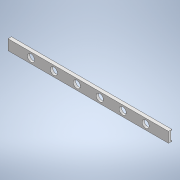
# Autodesk Inventor part: couvercle
Saved by Autodesk Inventor 2020 (Build 240168000, 168)
## iProperties
Created: 2023-04-05
Part Number: couvercle
Material: Générique
Document SubType Name: Modeling
Designer: Admin
Density: 1 g/cm^3
Appearance: Par défaut
Author: Admin
Autodesk Inventor part; units mm, degrees
ref_plane "YZ Plane" through (0, 0, 0) normal (1, 0, 0) x (0, 1, 0)
ref_plane "XZ Plane" through (0, 0, 0) normal (0, 1, 0) x (-1, 0, 0)
ref_plane "XY Plane" through (0, 0, 0) normal (0, 0, 1) x (1, 0, 0)
sketch "Esquisse1" plane through (0, 0, 0) normal (0, 0, 1) x (1, 0, 0)
  line L0 (40, 3.9877) -> (-100, 3.9877)
  line L1 (-100, 3.9877) -> (-100, -4.0123)
  line L2 (-100, -4.0123) -> (40, -4.0123)
  line L3 (40, -4.0123) -> (40, 3.9877)
  circle A0 centre (0, 0) radius 3.125
  line L4 (15.1704, 0) -> (0, 0) construction
  circle A1 centre (-20, 0) radius 3.125
  circle A2 centre (-40, 0) radius 3.125
  circle A3 centre (-60, 0) radius 3.125
  circle A4 centre (-80, 0) radius 3.125
  circle A5 centre (20, 0) radius 3.125
  dimension "d0" = 8
  dimension "d1" = 140
  dimension "d2" = 40
  dimension "d3" = 6.25
  dimension "d6" = 20
  dimension "d13" = 20
  constraints: 10 end point, 6 centre point, 4 horizontal, 2 parallel, 1 coincident, 1 perpendicular, 10 other
  measures "d0" distance of L0.end L1.end
  measures "d1" distance of L1.end L2.end
  measures "d2" distance from line of point (0, 0) L3
  measures "d3" diameter of A0
  measures "d6" distance of L4.end A1.centre
  measures "d13" distance of L4.end A5.centre
extrude "Extrusion1" add sketch "Esquisse1" along normal blind 2
sketch "Esquisse2" plane through (0, 0, 2) normal (0, 0, 1) x (1, 0, 0)
  line L0 (-100, 3.9877) -> (40, 3.9877)
  line L1 (40, 3.9877) -> (40, 4.4877)
  line L2 (40, 4.4877) -> (-100, 4.4877)
  line L3 (-100, 4.4877) -> (-100, 3.9877)
  line L4 (40, -4.0123) -> (-100, -4.0123)
  line L5 (-100, -4.0123) -> (-100, -4.5123)
  line L6 (-100, -4.5123) -> (40, -4.5123)
  line L7 (40, -4.5123) -> (40, -4.0123)
  point P0 (0, 0)
  dimension "d20" = 140
  dimension "d21" = 140
  dimension "d22" = 0.5
  dimension "d23" = 0.5
  constraints: 16 end point, 4 parallel, 2 horizontal, 2 perpendicular
  measures "d20" distance of L2.end L1.end
  measures "d21" distance of L6.end L5.end
  measures "d22" distance of L0.end L1.end
  measures "d23" distance of L6.end L4.start
extrude "Extrusion2" add sketch "Esquisse2" against normal blind 3
